Autodesk Inventor part; units mm, degrees
(part 2 of 2)
  dimension "d65" = 2.5
  dimension "d89" = 6.6
  dimension "d96" = 6.6
  dimension "d103" = 11.43154
  dimension "d108" = 0.6
  dimension "d109" = 0.6
  dimension "d110" = 0.6
  dimension "d113" = 6.6
  dimension "d120" = 6.6
  dimension "d125" = 0.6
  dimension "d126" = 0.6
  dimension "d127" = 90
  dimension "d128" = 6
  constraints: 732 end point, 8 centre point, 8 point on circle, 5 symmetric about line, 4 coincident, 4 midpoint, 4 tangent, 2 point on line, 1 collinear, 1 parallel, 972 other
  measures "d1" diameter of A2
  measures "d2" radius of A3
  measures "d6" diameter of A6
  measures "d57" radius of A8
  measures "d89" distance of L7.end L14.start
  measures "d96" distance of L7.end L20.start
  measures "d103" distance of L8.end L26.start
  measures "d108" distance between parallel lines of L10 L15
  measures "d109" distance between parallel lines of L20 L5
  measures "d110" distance between parallel lines of L24 L28
  measures "d113" distance of L5.end L80.start
  measures "d120" distance of L5.start L176.start
  measures "d125" distance between parallel lines of L178 L6
  measures "d126" distance between parallel lines of L9 L80
  measures "d127" horizontal distance of L3.end A9.centre
  measures "d128" distance between parallel lines of L272 L275
extrude "押し出し1" add sketch "スケッチ2" along normal blind 11 contours L0 L130 L129 L128 L133 L132 A9 L135 L136 L137 L140 L142 L143 L98 L41 L42 L43 L38 L32 L33 L34 L35 L188 L242 L241 L240 L232 L231 L230 L224 L225 L226 L227 L228 L2 A5 L4 A3 | L0 A9 L132 L133 L128 L129 L130 | A8 L132 A9 | A8 L135 A9 L132 | L228 L227 L226 L225 L224 A9 L2 | A8 L138 L137 A10 A9 L135 | A9 A10 L136 L135 | A9 L224 A8 | A8 L334 L335 A10 L137 L138 | L224 A9 L230 A8 | A8 L337 L336 A10 L335 L334 | L137 A10 L335 L336 L147 L146 L151 L150 L149 L153 L152 L157 L156 L155 L154 L112 L111 L110 L115 L114 L117 L116 L63 L64 L214 L215 L211 L206 L207 L208 L209 L253 L252 L251 L250 L249 L248 L246 L245 L244 L236 L237 L291 L290 L232 A9 L240 L239 L238 L243 L242 L188 L189 L199 L198 L197 L196 L35 L36 L37 L32 L38 L39 L40 L41 L98 L103 L102 L101 L100 L99 L143 L144 L145 L141 L140 | L230 A9 A10 L232 L233 A8 | L230 L231 A10 A9 | A8 L349 L348 L347 L159 L158 L163 L118 L117 A10 L114 L113 L112 L154 L153 L149 L148 L147 L336 L337 | L233 L232 A10 L290 L289 A8 | A8 L347 L348 L349 | L289 L290 A10 L291 L286 A8 | L147 L148 L149 A10 | L286 L291 A10 L237 L247 L246 L248 L253 L209 L210 L211 L215 L213 A8 L254 L255 L256 L300 L299 L298 | A8 L163 L158 L159 | L298 L299 L300 A8 | L153 L154 A10 | A10 L246 L247 L237 | A8 L121 L116 A10 L117 L118 | L256 L255 L254 A8 | A8 L62 A10 L116 L121 | L112 L113 L114 A10 | A10 L253 L248 | A8 L65 A10 L62 | L213 L215 A10 L214 L216 A8 | A8 L216 L214 A10 L65 | A10 L211 L210 L209
extrude "押し出し2" add sketch "スケッチ2" along normal blind 10 contours A6 | A7
extrude "押し出し3" cut sketch "スケッチ2" along normal blind 1 contours A6 | A7
fillet "フィレット1" radius 2 12 edges at (-26.2641, 0, -108.9378) (-20.9321, 0, -120.9157) (-19.5608, 0, -133.9548) (-54.9645, 0, -145.5638) (-62.7291, 0, -116.586) (-26.2641, 11, -108.9378) (-20.9321, 11, -120.9157) (-19.5608, 11, -133.9548) (-54.9645, 11, -145.5638) (-62.7291, 11, -116.586) (-122.0965, 11, -148.0226) (-122.0965, 0, -148.0226)
fillet "フィレット2" radius 10 6 edges at (-86.5065, 10.4476, -153.3736) (-86.5065, 0.5524, -153.3736) (-86.1177, 5.5, -153.9113) (-93.8823, 5.5, -124.9335) (-93.9502, 0.5524, -125.5935) (-93.9502, 10.4476, -125.5935)
